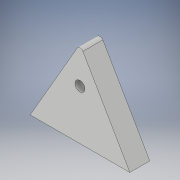
# Autodesk Inventor part: Rocker Base Joint
Saved by Autodesk Inventor 2019 (Build 230136000, 136)
## iProperties
Created: 2021-06-06
Part Number: Rocker Base Joint
Material: Generic
Document SubType Name: Modeling
Designer: micha
Density: 1 g/cm^3
Appearance: Default
Author: micha
Autodesk Inventor part; units mm, degrees
ref_plane "YZ Plane" through (0, 0, 0) normal (1, 0, 0) x (0, 1, 0)
ref_plane "XZ Plane" through (0, 0, 0) normal (0, 1, 0) x (-1, 0, 0)
ref_plane "XY Plane" through (0, 0, 0) normal (0, 0, 1) x (1, 0, 0)
sketch "Sketch1" plane through (0, 0, 0) normal (0, 0, 1) x (1, 0, 0)
  line L0 (0, 0) -> (-30, 0)
  line L1 (0, 0) -> (30, 0)
  line L2 (30, 0) -> (0, 51.9615)
  line L3 (0, 51.9615) -> (-30, 0)
  dimension "d0" = 30
  dimension "d1" = 30
  dimension "d2" = 60
  dimension "d3" = 60
  constraints: 8 end point, 2 horizontal
  measures "d0" distance of L0.start L0.end
  measures "d1" distance of L0.start L1.end
  measures "d2" distance of L1.end L2.end
  measures "d3" angle of L2 L1
extrude "Extrusion1" add sketch "Sketch1" along normal blind 12
sketch "Sketch2" plane through (0, 0, 12) normal (0, 0, 1) x (1, 0, 0)
  line L0 (0, 0) -> (0, 30)
  circle A0 centre (0, 30) radius 3
  dimension "d7" = 30
  dimension "d8" = 6
  constraints: 2 end point, 1 centre point, 1 coincident, 1 vertical
  measures "d7" distance of L0.start L0.end
  measures "d8" diameter of A0
extrude "Extrusion2" cut sketch "Sketch2" against normal through all
fillet "Fillet2" radius 2 1 edges at (0, 51.9615, 6)
body "Solid1"
